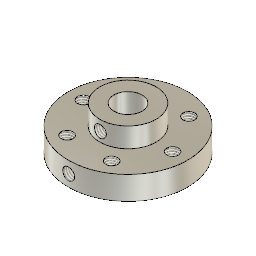
Mouting hub (Autodesk Fusion 360 design; units mm, degrees)
Autodesk Fusion 360 part; units mm, degrees
sketch "Esquisse1" plane through (0, 0, 0) normal (0, 0, 1) x (1, 0, 0)
  circle A0 centre (0, 0) radius 12.7
  circle A1 centre (0, 0) radius 6
  circle A2 centre (0, 0) radius 3
  dimension "d1" = 25.4
  dimension "d2" = 12
  dimension "d3" = 6
  constraint coincident A0.centre A1.centre
  constraint concentric A0 A2
  measures "d1" diameter of A0
  measures "d2" diameter of A1
  measures "d3" diameter of A2
extrude "Extrusion1" add sketch "Esquisse1" along normal blind 5 contours A0
extrude "Extrusion2" add sketch "Esquisse1" along normal blind 9.2 contours A1
sketch "Esquisse2" plane through (0, 0, 5) normal (0, 0, 1) x (-1, 0, 0)
  circle A0 centre (0, 0) radius 6
  circle A1 centre (0, 0) radius 12.7
  circle A2 centre (0, 0) radius 9.5
  circle A3 centre (-9.5, 0) radius 0.445
  circle A4 centre (-4.75, -8.2272) radius 0.445
  circle A5 centre (4.75, -8.2272) radius 0.445
  circle A6 centre (9.5, 0) radius 0.445
  circle A7 centre (4.75, 8.2272) radius 0.445
  circle A8 centre (-4.75, 8.2272) radius 0.445
  point P0 (-4.75, -8.2272)
  point P1 (4.75, -8.2272)
  point P2 (9.5, 0)
  point P3 (4.75, 8.2272)
  point P4 (-4.75, 8.2272)
  dimension "d8" = 19
  dimension "d10" = 0.89
  dimension "d12" = 360
  dimension "d13" = 0.89
  dimension "d14" = 0.89
  dimension "d15" = 0.89
  dimension "d16" = 0.89
  dimension "d17" = 0.89
  constraint concentric A0 A2
  constraint coincident A2 A3.centre
  constraint coincident P0 A4.centre
  constraint coincident P1 A5.centre
  constraint coincident P2 A6.centre
  constraint coincident P3 A7.centre
  constraint coincident P4 A8.centre
  measures "d8" diameter of A2
  measures "d10" diameter of A3
  measures "d13" diameter of A4
  measures "d14" diameter of A5
  measures "d15" diameter of A6
  measures "d16" diameter of A7
  measures "d17" diameter of A8
hole "Perçage1" at (4.75, 8.2272, 5) at (-4.75, 8.2272, 5) at (-9.5, 0, 5) at (-4.75, -8.2272, 5) at (4.75, -8.2272, 5) at (9.5, 0, 5) direction (0, 0, -1) diameter 2.529 depth 6 tip angle 118
thread "Filetage1" "ANSI Metric M Profile 3.0 M3x0.5 6H" thread offset 0 thread depth 7.4
sketch "Esquisse3" plane through (0, 0, 0) normal (0, 1, 0) x (1, 0, 0)
  circle A0 centre (0, -2.5) radius 0.445
  circle A1 centre (0, -7) radius 0.445
  dimension "d23" = 0.89
  dimension "d24" = 0.89
  measures "d23" diameter of A0
  measures "d24" diameter of A1
hole "Perçage2" at (0, 0, 7) at (0, 0, 2.5) direction (0, -1, 0) diameter 2.529 depth 22.5 tip angle 118
thread "Filetage2" "ANSI Metric M Profile 3.0 M3x0.5 6H" thread offset 0 thread depth 7.4
